Axe (Autodesk Fusion 360 design; units mm, degrees)
Autodesk Fusion 360 part; units mm, degrees
note: some values were not read from the file. Chosen so that the rebuilt part matches the saved one: which face or edge a step refers to. Set by a fixed rule: which sketch regions a step uses.
sketch "Sketch1" plane through (0, 0, 0) normal (0, 0, 1) x (1, 0, 0)
  circle A0 centre (0, 0) radius 4
  circle A1 centre (0, 0) radius 5
  dimension "d2" = 8
  dimension "d11" = 1
  constraint coincident A0.centre A1.centre
  measures "d2" diameter of A0
extrude "Extrude1" add sketch "Sketch1" against normal blind 96 contours A0 | A1 makes body 1
extrude "Extrude12" cut sketch "Sketch1" against normal blind 7.2 bodies 1
sketch "Sketch3" plane through (0, 0, 0) normal (0, 0, 1) x (-1, 0, 0)
  line L0 (-2.8284, 2.8284) -> (2.8284, 2.8284)
  line L1 (2.8284, 2.8284) -> (2.8284, -2.8284)
  line L2 (2.8284, -2.8284) -> (-2.8284, -2.8284)
  line L3 (-2.8284, -2.8284) -> (-2.8284, 2.8284)
  line L4 (-2.8284, 2.8284) -> (2.8284, -2.8284) construction
  line L5 (2.8284, 2.8284) -> (-2.8284, -2.8284) construction
  circle A0 centre (0, 0) radius 4
  dimension "d14" = 5.6569
  dimension "d15" = 5.6569
  constraint perpendicular L0 L1
  constraint parallel L0 L2
  constraint parallel L1 L3
  constraint horizontal L0
  constraint coincident L4 A0.centre
  constraint coincident L5 A0.centre
  constraint coincident A0.centre origin
  constraint perpendicular L4 L5
  measures "d14" distance of L1.end L2.end
  measures "d15" distance of L0.end L1.end
extrude "Extrude5" add sketch "Sketch3" along normal blind 2 contours L0 L1 L2 L3 bodies 1
sketch "Sketch2" plane through (0, 0, -96) normal (0, 0, -1) x (1, 0, 0)
  circle A0 centre (0, 0) radius 2.65
  line L0 (-1.1236, 2.4) -> (1.1236, 2.4)
  circle A1 centre (0, 0) radius 5
  dimension "d7" = 5.3
  dimension "d8" = 2.4
  constraint coincident A0 L0.start
  constraint coincident A0 L0.end
  constraint horizontal L0
  measures "d7" diameter of A0
  measures "d8" distance of A0.centre L0
extrude "Extrude3" cut sketch "Sketch2" against normal blind 20 contours A0 L0 picked at (-0.0646, 0.673) bodies 1
sketch "Sketch4" plane through (0, 0, 2) normal (0, 0, 1) x (-1, 0, 0)
  circle A0 centre (0, 0) radius 0.75
  dimension "d19" = 1.5
  constraint coincident A0.centre origin
  measures "d19" diameter of A0
extrude "Extrude6" cut sketch "Sketch4" against normal blind 15 bodies 1
sketch "Sketch9" plane through (0, 0, 0) normal (0, 0, 1) x (1, 0, 0)
  circle A0 centre (0, 0) radius 29
  line L0 (2.9, 2.9) -> (-2.9, 2.9)
  line L1 (-2.9, 2.9) -> (-2.9, -2.9)
  line L2 (-2.9, -2.9) -> (2.9, -2.9)
  line L3 (2.9, -2.9) -> (2.9, 2.9)
  line L4 (2.9, 2.9) -> (-2.9, -2.9) construction
  line L5 (-2.9, 2.9) -> (2.9, -2.9) construction
  dimension "d40" = 58
  dimension "d41" = 5.8
  dimension "d42" = 5.8
  constraint coincident A0.centre origin
  constraint perpendicular L0 L1
  constraint parallel L0 L2
  constraint parallel L1 L3
  constraint horizontal L0
  constraint coincident L4 A0.centre
  constraint coincident L5 A0.centre
  measures "d40" diameter of A0
  measures "d41" distance of L1.end L2.end
  measures "d42" distance of L0.end L1.end
sketch "Sketch1 (2)" plane through (0, 0, 0) normal (0, 0, 1) x (1, 0, 0) in component "Bague Sup"
  circle A0 centre (0, 0) radius 4
  circle A1 centre (0, 0) radius 2.1
  dimension "d58" = 8
  dimension "d59" = 4.2
  constraint coincident A0.centre A1.centre
  constraint concentric A0 A1
  measures "d58" diameter of A0
  measures "d59" diameter of A1
extrude "Extrude1'" add sketch "Sketch1 (2)" along normal blind 6 separate body makes body 2 in component "Bague Sup"
move_body "Move1" bodies 2 to x (1, 0, 0) y (0, 1, 0) z (0, 0, 1) at (0, 70, 0) in component "Bague Sup"
extrude "Extrude10" add sketch "Sketch9" along normal blind 2 separate body makes body 3
sketch "Sketch5" plane through (0, 0, 2) normal (0, 0, 1) x (-1, 0, 0)
  line L0 (-2.9, -2.9) -> (-2.9, 2.9)
  line L1 (-2.9, 2.9) -> (-2.755, 2.9)
  arc A0 (-2.755, 2.9) -> (-2.8284, 2.8284) centre (0, 0) ccw
  line L2 (-2.8284, 2.8284) -> (2.8284, 2.8284)
  arc A1 (2.8284, 2.8284) -> (2.755, 2.9) centre (0, 0) ccw
  line L3 (2.755, 2.9) -> (2.9, 2.9)
  line L4 (2.9, 2.9) -> (2.9, -2.9)
  line L5 (2.9, -2.9) -> (2.755, -2.9)
  arc A2 (2.755, -2.9) -> (2.8284, -2.8284) centre (0, 0) ccw
  arc A3 (-2.8284, -2.8284) -> (-2.755, -2.9) centre (0, 0) ccw
  line L6 (-2.755, -2.9) -> (-2.9, -2.9)
  circle A4 centre (0, 0) radius 29
  line L7 (28.892, -2.5) -> (28.892, 2.5)
  line L8 (28.892, 2.5) -> (0, 0)
  line L9 (0, 0) -> (28.892, -2.5)
  circle A5 centre (0, 0) radius 16.1
  line L10 (-2.9, -2.9) -> (-2.9, 2.9)
  line L11 (-2.9, 2.9) -> (2.9, 2.9)
  line L12 (2.9, 2.9) -> (2.9, -2.9)
  line L13 (2.9, -2.9) -> (-2.9, -2.9)
  circle A6 centre (0, 0) radius 29
  line L14 (16.03, 1.5) -> (16.03, -1.5)
  line L15 (-16.03, -1.5) -> (-16.03, 1.5)
  line L16 (-16.03, 1.5) -> (16.03, -1.5) construction
  line L17 (16.03, 1.5) -> (-16.03, -1.5) construction
  line L18 (28.892, 2.5) -> (16.03, 1.3871)
  line L19 (28.892, -2.5) -> (16.0401, -1.3879)
  line L20 (16.03, -1.5) -> (2.9, -1.5)
  line L21 (-2.9, -1.5) -> (-16.03, -1.5)
  line L22 (-16.03, 1.5) -> (-2.9, 1.5)
  line L23 (2.9, 1.5) -> (16.03, 1.5)
  line L24 (9.465, -1.5) -> (9.465, 1.5)
  line L25 (-9.465, -1.5) -> (-9.465, 1.5)
  arc A7 (17.0363, 1.4741) -> (17.0363, -1.4741) centre (0, 0) ccw
  dimension "d24" = 5
  dimension "d35" = 32.2
  dimension "d49" = 3
  dimension "d52" = 3
  constraint coincident A4 L7.start
  constraint coincident A4 L7.end
  constraint parallel L4 L7
  constraint coincident A0.centre A1.centre
  constraint perpendicular L14 L22
  constraint parallel L20 L22
  constraint parallel L14 L15
  constraint horizontal L22
  constraint coincident A5 L15.end
  constraint coincident L16 A0.centre
  constraint coincident L17 A0.centre
  constraint coincident L8 L18.end
  constraint coincident L14 L18.end
  constraint coincident A5 L19.end
  constraint coincident L9 L19.end
  constraint coincident L4 L20.end
  constraint coincident L0 L21.start
  constraint collinear L20 L21
  constraint coincident L0 L22.end
  constraint coincident L4 L23.start
  constraint collinear L22 L23
  constraint midpoint L20 L24.start
  constraint midpoint L23 L24.end
  constraint midpoint L21 L25.start
  constraint midpoint L22 L25.end
  constraint concentric A5 A7
  constraint coincident L9 A7.end
  constraint coincident L8 A7.start
  measures "d24" distance of L7.start L7.end
  measures "d35" diameter of A5
  measures "d49" distance of L15.end L15.start
  measures "d52" distance of L20 L23
extrude "Extrude7" add sketch "Sketch5" along normal blind 9 contours L7 L8 L9 A5 L18 L19 | A4 L7 A6 bodies 3
extrude "Extrude13" add sketch "Sketch5" along normal blind 2 contours L15 L21 L22 L25 | L8 L9 A5 L18 L19 A7 | L9 L14 L20 L24 | L8 L14 L23 L24 | L8 L9 L14 L24 bodies 3
sketch "Sketch11" plane through (0, 0, 0) normal (0, 1, 0) x (1, 0, 0)
  circle A0 centre (-25.2661, -6.5) radius 2.6
  line L0 (-28.892, -6.5) -> (-16.0401, -6.5) construction
  circle A1 centre (-19.6661, -6.5) radius 2.6
  line L1 (-17.0363, -4) -> (-16.0401, -4)
  line L2 (-16.0401, -4) -> (-16.0401, -11)
  line L3 (-16.0401, -11) -> (-28.892, -11)
  line L4 (-28.892, -11) -> (-28.892, -2)
  line L5 (-28.892, -2) -> (-17.0363, -2)
  line L6 (-17.0363, -2) -> (-17.0363, -4)
  point P0 (-22.4661, -6.5)
  dimension "d54" = 5.2
  dimension "d55" = 5.2
  dimension "d56" = 2.8
  dimension "d57" = 2.8
  constraint coincident A0.centre L0
  constraint coincident A1.centre L0
  constraint midpoint P0 L0
  constraint midpoint L0.start L4
  constraint coincident L0.end L2
  constraint perpendicular L0 L2
  measures "d54" diameter of A0
  measures "d55" diameter of A1
  measures "d56" distance of P0 A0.centre
  measures "d57" distance of P0 A1.centre
extrude "Extrude9" cut sketch "Sketch11" along normal mid plane 5 contours A0 | A1 bodies 3
sketch "Sketch1 (3)" plane through (0, 0, 0) normal (0, 0, 1) x (1, 0, 0) in component "Connexion_Moteur"
  circle A0 centre (0, 0) radius 2.65
  line L0 (-1.1236, 2.4) -> (1.1236, 2.4)
  circle A1 centre (0, 0) radius 4
  circle A2 centre (0, 0) radius 2.1
  dimension "d62" = 5.3
  dimension "d63" = 2.4
  dimension "d64" = 8
  dimension "d67" = 4.2
  constraint coincident A0.centre A1.centre
  constraint coincident A0 L0.start
  constraint coincident A0 L0.end
  constraint horizontal L0
  constraint concentric A0 A2
  measures "d62" diameter of A0
  measures "d63" distance of A0.centre L0
  measures "d64" diameter of A1
  measures "d67" diameter of A2
extrude "Extrude1''" add sketch "Sketch1 (3)" against normal blind 15 separate body contours A0 L0 | A1 picked at (0.1285, 2.4739) makes body 4 in component "Connexion_Moteur"
extrude "Extrude2" add sketch "Sketch1 (3)" along normal blind 15 contours A0 L0 | A0 L0 | A1 bodies 4 in component "Connexion_Moteur"
sketch "Sketch1 (4)" plane through (0, 0, 0) normal (0, 0, 1) x (1, 0, 0) in component "Tige_Filtée_4"
  circle A0 centre (0, 0) radius 2
  dimension "d70" = 4
  constraint coincident A0.centre origin
  measures "d70" diameter of A0
extrude "Extrude1'''" add sketch "Sketch1 (4)" along normal blind 90 separate body makes body 5 in component "Tige_Filtée_4"
move_face "MoveFace1" to x (1, 0, 0) y (0, 1, 0) z (0, 0, 1) at (-55, 0, 0) 1 faces at (1.9975, -0.0997, 60) on bodies 5 in component "Tige_Filtée_4"
sketch "Sketch1 (5)" plane through (0, 0, 0) normal (0, 0, 1) x (-1, 0, 0) in component "Entretoise M4"
  circle A0 centre (0, 0) radius 7.5
  line L0 (-2.0785, 3.6) -> (-4.1569, 0)
  line L1 (-4.1569, 0) -> (-2.0785, -3.6)
  line L2 (-2.0785, -3.6) -> (2.0785, -3.6)
  line L3 (2.0785, -3.6) -> (4.1569, 0)
  line L4 (4.1569, 0) -> (2.0785, 3.6)
  line L5 (2.0785, 3.6) -> (-2.0785, 3.6)
  circle A1 centre (0, 0) radius 2.25
  dimension "d73" = 7.2
  dimension "d74" = 15
  dimension "d75" = 4.5
  constraint coincident A0.centre A1.centre
  constraint concentric A0 A1
  measures "d73" distance of L2 L5
  measures "d74" diameter of A0
  measures "d75" diameter of A1
extrude "Extrude4" add sketch "Sketch1 (5)" along normal mid plane 20 separate body contours A0 | L0 L1 L2 L3 L4 L5 makes body 6 in component "Entretoise M4"
extrude "Extrude5'" cut sketch "Sketch1 (5)" along normal mid plane 12 contours L0 L1 L2 L3 L4 L5 bodies 6 in component "Entretoise M4"
sketch "Sketch5 (2)" plane through (0, 0, 0) normal (0, 1, 0) x (1, 0, 0) in component "Entretoise M4"
  line L0 (4.1569, 4) -> (-4.1569, 4)
  line L1 (-4.1569, 4) -> (-4.1569, -4)
  line L2 (-4.1569, -4) -> (4.1569, -4)
  line L3 (4.1569, -4) -> (4.1569, 4)
  line L4 (4.1569, 4) -> (-4.1569, -4) construction
  line L5 (-4.1569, 4) -> (4.1569, -4) construction
  line L6 (-4.1569, -6) -> (-4.1569, 6)
  line L7 (-4.1569, 6) -> (-2.0785, 6)
  line L8 (-2.0785, 6) -> (-2.0785, -6)
  line L9 (-2.0785, -6) -> (-4.1569, -6)
  line L10 (2.0785, -6) -> (2.0785, 6)
  line L11 (2.0785, 6) -> (4.1569, 6)
  line L12 (4.1569, 6) -> (4.1569, -6)
  line L13 (4.1569, -6) -> (2.0785, -6)
  dimension "d87" = 8
  constraint perpendicular L0 L1
  constraint parallel L0 L2
  constraint parallel L1 L3
  constraint horizontal L0
  constraint coincident L4 origin
  constraint coincident L5 origin
  constraint coincident L0.end L6
  measures "d87" distance of L0.end L1.end
extrude "Extrude6'" cut sketch "Sketch5 (2)" along normal blind 10.5 contours L0 L2 L3 L10 L12 | L0 L2 L8 L10 | L0 L1 L2 L6 L8 bodies 6 in component "Entretoise M4"
component "Bague Sup" placed x (1, 0, 0) y (0, 1, 0) z (0, 0, 1) at (0, 0, 0)
component "Connexion_Moteur" placed x (1, 0, 0) y (0, 1, 0) z (0, 0, 1) at (0, 50, 0)
component "Tige_Filtée_4" placed x (1, 0, 0) y (0, 1, 0) z (0, 0, 1) at (0, 0, 0)
component "Entretoise M4" placed x (1, 0, 0) y (0, 1, 0) z (0, 0, 1) at (0, 0, 0)
hidden bodies 1
named bodies: "Axe", "Plate", "Bague Sup", "Connexion_Moteur"
